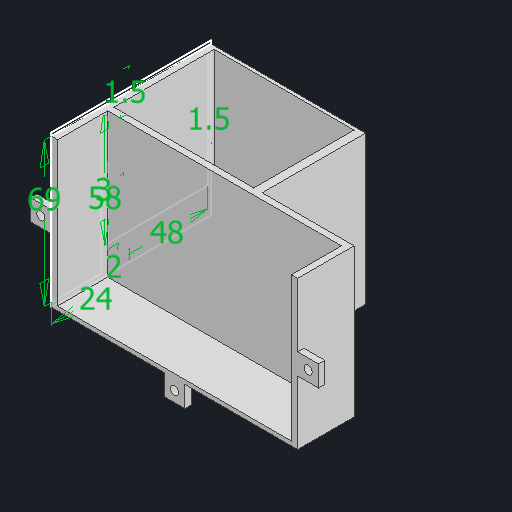
# Autodesk Inventor part: battery_base
Saved by Autodesk Inventor 2026.1 (Build 301233020, 233B)
## iProperties
Created: 2025-11-26
Part Number: battery_base
Material: 일반
Document SubType Name: Modeling
Designer: jaewook
Density: 1 g/cm^3
Appearance: 기본값
Author: jaewook
Autodesk Inventor part; units mm, degrees
ref_plane "YZ Plane" through (0, 0, 0) normal (1, 0, 0) x (0, 1, 0)
ref_plane "XZ Plane" through (0, 0, 0) normal (0, 1, 0) x (-1, 0, 0)
ref_plane "XY Plane" through (0, 0, 0) normal (0, 0, 1) x (1, 0, 0)
sketch "스케치1" plane through (0, 0, 0) normal (1, 0, 0) x (0, 1, 0)
  line L0 (0, 0) -> (72.5, 0)
  line L1 (72.5, 0) -> (72.5, -76.5)
  line L2 (72.5, -76.5) -> (0, -76.5)
  line L3 (0, -76.5) -> (0, 0)
  line L4 (2, -24) -> (71, -24)
  line L5 (71, -24) -> (71, 0)
  line L6 (71, 0) -> (2, 0)
  line L7 (2, 0) -> (2, -24)
  line L8 (13, -75) -> (71, -75)
  line L9 (71, -75) -> (71, -27)
  line L10 (71, -27) -> (13, -27)
  line L11 (13, -27) -> (13, -75)
  line L12 (71, -27) -> (71, -24)
  line L13 (71, -75) -> (71, -76.5)
  point P0 (71, 0)
  point P1 (2, 0)
  dimension "d1" = 69
  dimension "d3" = 58
  dimension "d4" = 1.5
  dimension "d5" = 3
  dimension "d6" = 24
  dimension "d7" = 48
  dimension "d8" = 1.5
  dimension "d9" = 2
  constraints: 28 end point, 6 parallel, 5 perpendicular, 3 horizontal, 2 collinear, 1 point on line
  measures "d1" distance of L5.end L6.end
  measures "d3" distance of L9.end L10.end
  measures "d4" distance between parallel lines of L1 L5
  measures "d5" distance between parallel lines of L4 L10
  measures "d6" distance of L6.end L4.start
  measures "d7" distance of L10.end L8.start
  measures "d8" distance between parallel lines of L8 L2
  measures "d9" distance between parallel lines of L3 L7
extrude "돌출1" add sketch "스케치1" along normal blind 118 contours L0 L7 L4 L12 L10 L11 L8 L13 L2 L3 | L0 L5 L4 L7 | L8 L11 L10 L9
extrude "돌출2" cut sketch "스케치1" along normal blind 70 contours L8 L11 L10 L9
extrude "돌출3" cut sketch "스케치1" along normal blind 115 contours L0 L5 L4 L7
sketch "스케치2" plane through (0, 71, -76.5) normal (0, 1, 0) x (1, 0, 0)
  line L0 (118, 0) -> (118, -76.5) projected
  line L1 (0, 0) -> (118, 0) projected
  line L2 (70, -1.5) -> (70, -49.5) projected
  line L3 (70, -49.5) -> (0, -49.5) projected
  line L4 (74, 0) -> (118, 0)
  line L5 (118, 0) -> (118, -49.5)
  line L6 (118, -49.5) -> (74, -49.5)
  line L7 (74, -49.5) -> (74, 0)
  point P0 (0, -76.5)
  dimension "d16" = 4
  constraints: 8 end point, 2 parallel, 2 point on line, 1 collinear, 1 horizontal, 1 perpendicular
  measures "d16" distance between parallel lines of L7 L2
extrude "돌출4" cut sketch "스케치2" against normal blind 113
sketch "스케치3" plane through (0, 0, 0) normal (-1, 0, 0) x (0, 0, 1)
  line L0 (0, 2) -> (-24, 2) projected
  line L1 (-24, 2) -> (-24, 71) projected
  line L2 (-27, 71) -> (-27, 13) projected
  line L3 (-27, 13) -> (-75, 13) projected
  line L4 (-75, 13) -> (-75, 71) projected
  line L5 (-24, 71) -> (0, 71) projected
  line L6 (0, 2) -> (0, 71)
  line L7 (0, 71) -> (-24, 71)
  line L8 (-24, 71) -> (-75, 71)
  constraints: 6 end point, 1 collinear, 1 perpendicular, 1 vertical
extrude "돌출5" add sketch "스케치3" against normal blind 3
sketch "스케치4" plane through (0, 0, 0) normal (0, 0, 1) x (1, 0, 0)
  line L0 (0, 71) -> (0, 0) projected
  line L1 (0, 0) -> (118, 0) projected
  line L2 (118, 71) -> (118, 0) projected
  line L3 (118, 71) -> (0, 71)
  line L4 (0, 0) -> (74, 0) projected
  line L5 (59, 0) -> (59, 71) construction
  line L6 (118, 35.5) -> (0, 35.5) construction
  line L7 (118, 40.5) -> (128, 40.5)
  line L8 (128, 40.5) -> (128, 30.5)
  line L9 (128, 30.5) -> (118, 30.5)
  line L10 (118, 30.5) -> (118, 40.5)
  circle A0 centre (123, 35.5) radius 2
  line L11 (54, 0) -> (64, 0)
  line L12 (64, 0) -> (64, -10)
  line L13 (64, -10) -> (54, -10)
  line L14 (54, -10) -> (54, 0)
  circle A1 centre (59, -5) radius 2
  line L15 (-10, 40.5) -> (0, 40.5)
  line L16 (0, 40.5) -> (0, 30.5)
  line L17 (0, 30.5) -> (-10, 30.5)
  line L18 (-10, 30.5) -> (-10, 40.5)
  circle A2 centre (-5, 35.5) radius 2
  point P0 (54, 0)
  dimension "d21" = 10
  dimension "d22" = 10
  dimension "d23" = 4
  dimension "d24" = 5
  dimension "d25" = 5
  dimension "d26" = 10
  dimension "d27" = 10
  dimension "d28" = 4
  dimension "d29" = 5
  dimension "d30" = 5
  dimension "d31" = 10
  dimension "d32" = 10
  dimension "d33" = 4
  dimension "d34" = 5
  dimension "d35" = 5
  dimension "d38" = 40.5
  dimension "d39" = 128
  constraints: 30 end point, 6 parallel, 5 horizontal, 3 centre point, 3 midpoint, 3 perpendicular, 2 collinear, 2 point on line, 1 vertical, 3 other
  measures "d21" distance of L8.end L9.end
  measures "d22" distance of L7.end L8.end
  measures "d23" diameter of A0
  measures "d24" distance from line of L9 A0.centre
  measures "d25" distance from line of L8 A0.centre
  measures "d26" distance of L12.end L14.start
  measures "d27" distance of L11.end L12.end
  measures "d28" diameter of A1
  measures "d29" distance from line of L13 A1.centre
  measures "d30" distance from line of L12 A1.centre
  measures "d31" distance of L16.end L18.start
  measures "d32" distance of L15.end L16.end
  measures "d33" diameter of A2
  measures "d34" distance from line of L17 A2.centre
  measures "d35" distance from line of L16 A2.centre
  measures "d38" vertical distance of A2.centre A1.centre
  measures "d39" distance of A2.centre A0.centre
extrude "돌출6" add sketch "스케치4" against normal blind 3 contours L0 L17 L18 L15 | L7 L8 L9 L2 | L1 L12 L13 L14
